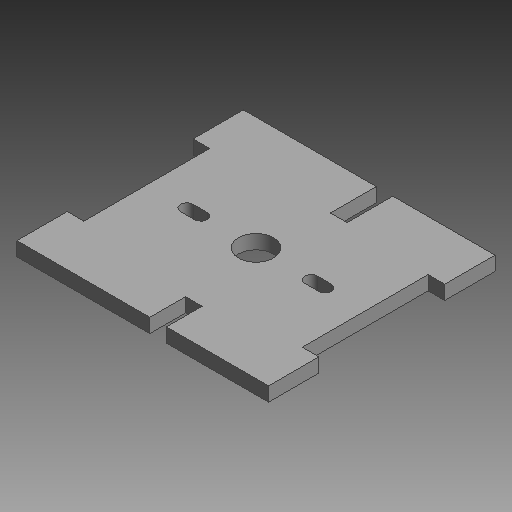
# Autodesk Inventor part: Part12
Saved by Autodesk Inventor 2019.2 (Build 232265000, 265)
## iProperties
Part Number: Part12
Material: Generic
Document SubType Name: Modeling
Designer: richard.girt
Mass: 5.51387 g
Surface Area: 47.3507 cm^2
Volume: 5.51387 cm^3
Density: 1 g/cm^3
Appearance: Default
Author: richard.girt
Autodesk Inventor part; units mm, degrees
ref_plane "YZ Plane" through (0, 0, 0) normal (1, 0, 0) x (0, 1, 0)
ref_plane "XZ Plane" through (0, 0, 0) normal (0, 1, 0) x (-1, 0, 0)
ref_plane "XY Plane" through (0, 0, 0) normal (0, 0, 1) x (1, 0, 0)
sketch "Sketch1" plane through (0, 0, 0) normal (0, 1, 0) x (-1, 0, 0)
  line L0 (-25, 22.5) -> (25, 22.5)
  line L1 (25, 22.5) -> (25, -22.5)
  line L2 (25, -22.5) -> (-25, -22.5)
  line L3 (-25, -22.5) -> (-25, 22.5)
  line L4 (-25, 22.5) -> (25, -22.5) construction
  line L5 (25, 22.5) -> (-25, -22.5) construction
  line L6 (25, -12.5) -> (21.7, -12.5)
  line L7 (21.7, -12.5) -> (21.7, 12.5)
  line L8 (21.7, 12.5) -> (25, 12.5)
  line L9 (25, 12.5) -> (25, -12.5)
  line L10 (-25, -12.5) -> (-21.7, -12.5)
  line L11 (-21.7, -12.5) -> (-21.7, 12.5)
  line L12 (-21.7, 12.5) -> (-25, 12.5)
  line L13 (-25, 12.5) -> (-25, -12.5)
  line L14 (-1.4, -22.5) -> (-4.7, -22.5)
  line L15 (-4.7, -22.5) -> (-4.7, -13.4)
  line L16 (-4.7, -13.4) -> (-1.4, -13.4)
  line L17 (-1.4, -13.4) -> (-1.4, -22.5)
  line L18 (-1.4, 22.5) -> (-4.7, 22.5)
  line L19 (-4.7, 22.5) -> (-4.7, 15.4)
  line L20 (-4.7, 15.4) -> (-1.4, 15.4)
  line L21 (-1.4, 15.4) -> (-1.4, 22.5)
  circle A0 centre (0, 0) radius 3.5
  line L22 (15, 0) -> (9.7, 0) construction
  line L23 (13.75, -1.25) -> (10.95, -1.25)
  line L24 (10.95, 1.25) -> (13.75, 1.25)
  arc A1 (13.75, -1.25) -> (13.75, 1.25) centre (13.75, 0) ccw
  arc A2 (10.95, 1.25) -> (10.95, -1.25) centre (10.95, 0) ccw
  line L25 (-9.7, 0) -> (-15, 0) construction
  line L26 (-10.95, -1.25) -> (-13.75, -1.25)
  line L27 (-13.75, 1.25) -> (-10.95, 1.25)
  arc A3 (-10.95, -1.25) -> (-10.95, 1.25) centre (-10.95, 0) ccw
  arc A4 (-13.75, 1.25) -> (-13.75, -1.25) centre (-13.75, 0) ccw
  line L28 (9.7, 0) -> (0, 0) construction
  line L29 (-9.7, 0) -> (0, 0) construction
  point P0 (21.7, 0)
  point P1 (12.35, 0)
  point P2 (-12.35, 0)
  dimension "d0" = 45
  dimension "d1" = 50
  dimension "d2" = 3.3
  dimension "d3" = 25
  dimension "d4" = 9.1
  dimension "d5" = 20.3
  dimension "d6" = 7
  dimension "d7" = 5.3
  dimension "d8" = 2.5
  dimension "d9" = 30
  dimension "d12" = 7.1
  constraints: 64 end point, 17 equal length, 14 point on line, 12 point on circle, 8 tangent, 7 horizontal, 7 midpoint, 5 centre point, 5 perpendicular, 3 horizontal alignment, 1 coincident, 1 equal radius
  measures "d0" distance of L0.end L1.end
  measures "d1" distance of L1.end L2.end
  measures "d2" distance of L11.end L12.end
  measures "d3" distance of L10.end L11.end
  measures "d4" distance of L14.end L15.end
  measures "d5" distance between parallel lines of L3 L15
  measures "d6" diameter of A0
  measures "d7" distance of L22.start L22.end
  measures "d8" distance between parallel lines of L26 L27
  measures "d9" distance of L22.start L25.end
  measures "d12" distance of L18.end L19.end
extrude "Extrusion1" add sketch "Sketch1" along normal blind 2.8 contours L0 L19 L20 L21 L1 L8 L7 L6 L2 L17 L16 L15 L3 L10 L11 L12
body "Solid1"
